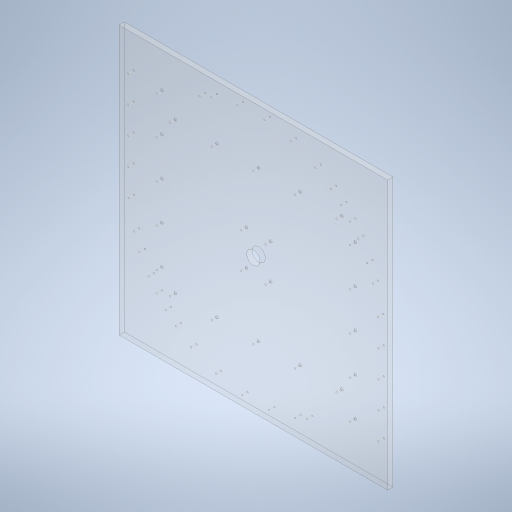
# Autodesk Inventor part: groundPlateWoodV1
Saved by Autodesk Inventor 2024.4 (Build 284460000, 460)
## iProperties
Created: 2025-11-05
Part Number: groundPlateWoodV1
Material: PMMA Plastic
Document SubType Name: Modeling
Designer: jonas
Density: 1.188 g/cm^3
Appearance: Polycarbonate - Clear
Author: jonas
Autodesk Inventor part; units mm, degrees
ref_plane "YZ Plane" through (0, 0, 0) normal (1, 0, 0) x (0, 1, 0)
ref_plane "XZ Plane" through (0, 0, 0) normal (0, 1, 0) x (-1, 0, 0)
ref_plane "XY Plane" through (0, 0, 0) normal (0, 0, 1) x (1, 0, 0)
sketch "Sketch1" plane through (0, 0, 0) normal (0, 1, 0) x (-1, 0, 0)
  line L0 (0, -102.1042) -> (0, 102.1042) construction
  line L1 (37.5532, 0) -> (-37.5532, 0) construction
  line L2 (500, 500) -> (-500, 500)
  line L3 (-500, 500) -> (-500, -500)
  line L4 (-500, -500) -> (500, -500)
  line L5 (500, -500) -> (500, 500)
  circle A0 centre (0, 0) radius 25
  dimension "d0" = 1000
  dimension "d1" = 1000
  dimension "d2" = 50
  constraints: 12 end point, 2 coincident, 2 horizontal, 2 midpoint, 2 parallel, 1 centre point, 1 perpendicular, 1 vertical, 2 other
  measures "d0" distance between parallel lines of L2 L4
  measures "d1" distance between parallel lines of L3 L5
  measures "d2" diameter of A0
extrude "Extrusion1" add sketch "Sketch1" along normal blind 20
sketch "Sketch3" plane through (0, 20, 0) normal (0, 1, 0) x (1, 0, 0)
  line L0 (464.3817, -39.9852) -> (0, 0) construction
  line L1 (0, 0) -> (445.1648, -138.1214) construction
  line L2 (423.7332, -194.1633) -> (0, 0) construction
  line L3 (360.2723, -295.7246) -> (0, 0) construction
  line L4 (289.0138, -365.6778) -> (0, 0) construction
  line L5 (389.8771, -255.4312) -> (0, 0) construction
  line L6 (326.5218, -332.615) -> (0, 0) construction
  line L7 (230.9911, -404.8361) -> (0, 0) construction
  line L8 (139.32, -444.7911) -> (0, 0) construction
  line L9 (41.2359, -464.2723) -> (0, 0) construction
  line L10 (464.3817, -39.9852) -> (445.1648, -138.1214) construction
  line L11 (445.1648, -138.1214) -> (423.7332, -194.1633) construction
  line L12 (423.7332, -194.1633) -> (389.8771, -255.4312) construction
  line L13 (389.8771, -255.4312) -> (360.2723, -295.7246) construction
  line L14 (360.2723, -295.7246) -> (326.5218, -332.615) construction
  line L15 (326.5218, -332.615) -> (289.0138, -365.6778) construction
  line L16 (289.0138, -365.6778) -> (230.9911, -404.8361) construction
  line L17 (230.9911, -404.8361) -> (139.32, -444.7911) construction
  line L18 (139.32, -444.7911) -> (41.2359, -464.2723) construction
  line L19 (-58.7462, -462.3831) -> (0, 0) construction
  line L20 (-156.0243, -439.2102) -> (0, 0) construction
  line L21 (-200, -421.0098) -> (0, 0) construction
  line L22 (41.2359, -464.2723) -> (-58.7462, -462.3831) construction
  line L23 (-58.7462, -462.3831) -> (-156.0243, -439.2102) construction
  line L24 (-200, -421.0098) -> (-156.0243, -439.2102) construction
  line L25 (500, 500) -> (-500, 500) projected
  line L26 (500, -500) -> (500, 500) projected
  line L27 (-16.3542, 0) -> (16.3542, 0) construction
  line L28 (0, 9.5055) -> (0, -9.5055) construction
  line L29 (-500, -500) -> (500, -500) projected
  line L30 (-466.1, -260) -> (-466.1, -360) construction
  line L31 (-500, 500) -> (-500, -500) construction
  line L32 (-466.1, -260) -> (-466.1, -160) construction
  line L33 (-466.1, -160) -> (-466.1, -60) construction
  line L34 (-464.3817, 39.9852) -> (0, 0) construction
  line L35 (-445.1648, 138.1214) -> (0, 0) construction
  circle A0 centre (0, 0) radius 25 construction
  line L36 (-423.7332, 194.1633) -> (0, 0) construction
  line L37 (0, 0) -> (-389.8771, 255.4312) construction
  line L38 (-360.2723, 295.7246) -> (0, 0) construction
  line L39 (-326.5218, 332.615) -> (0, 0) construction
  line L40 (0, 0) -> (-289.0138, 365.6778) construction
  line L41 (-230.9911, 404.8361) -> (0, 0) construction
  line L42 (-139.32, 444.7911) -> (0, 0) construction
  line L43 (-41.2359, 464.2723) -> (0, 0) construction
  line L44 (-466.1, -60) -> (-464.3817, 39.9852) construction
  line L45 (-464.3817, 39.9852) -> (-445.1648, 138.1214) construction
  line L46 (-445.1648, 138.1214) -> (-423.7332, 194.1633) construction
  line L47 (-423.7332, 194.1633) -> (-389.8771, 255.4312) construction
  line L48 (-389.8771, 255.4312) -> (-360.2723, 295.7246) construction
  line L49 (-360.2723, 295.7246) -> (-326.5218, 332.615) construction
  line L50 (-326.5218, 332.615) -> (-289.0138, 365.6778) construction
  line L51 (-289.0138, 365.6778) -> (-230.9911, 404.8361) construction
  line L52 (-230.9911, 404.8361) -> (-139.32, 444.7911) construction
  line L53 (-139.32, 444.7911) -> (-41.2359, 464.2723) construction
  line L54 (58.7462, 462.3831) -> (0, 0) construction
  line L55 (156.0243, 439.2102) -> (0, 0) construction
  line L56 (200, 421.0098) -> (0, 0) construction
  line L57 (58.7462, 462.3831) -> (-41.2359, 464.2723) construction
  line L58 (58.7462, 462.3831) -> (156.0243, 439.2102) construction
  line L59 (156.0243, 439.2102) -> (200, 421.0098) construction
  point P0 (466.1, 360)
  point P1 (466.1, 260)
  point P2 (466.1, 160)
  point P3 (466.1, 60)
  dimension "d62" = 100
  dimension "d63" = 100
  dimension "d64" = 100
  dimension "d66" = 466.1
  dimension "d67" = 100
  dimension "d68" = 100
  dimension "d69" = 60
  dimension "d70" = 70
  dimension "d71" = 50
  dimension "d72" = 70
  dimension "d73" = 100
  dimension "d76" = 140
  dimension "d77" = 33.9
  dimension "d78" = 700
  dimension "d79" = 140
  dimension "d80" = 100
  dimension "d82" = 33.9
  dimension "d84" = 60
  dimension "d85" = 70
  dimension "d86" = 50
  dimension "d87" = 70
  dimension "d88" = 100
  dimension "d89" = 700
  constraints: 112 end point, 39 equal length, 6 vertical alignment, 3 vertical, 2 midpoint, 1 coincident, 1 collinear, 1 horizontal
  measures "d62" distance of point (466.1, 260) point (466.1, 360)
  measures "d63" distance of point (466.1, 260) point (466.1, 160)
  measures "d64" distance of point (466.1, 160) point (466.1, 60)
  measures "d66" distance of L10.start L0.end
  measures "d67" distance of L10.start L11.start
  measures "d68" distance of point (466.1, 60) L10.start
  measures "d69" distance of L11.start L11.end
  measures "d70" distance of L11.end L13.start
  measures "d71" distance of L14.start L14.end
  measures "d72" distance of L17.start L15.end
  measures "d73" distance of L17.start L17.end
  measures "d76" distance from line of L25 point (466.1, 360)
  measures "d77" distance from line of L26 point (466.1, 360)
  measures "d78" distance from line of L26 L24.start
  measures "d79" distance from line of L29 L30.end
  measures "d80" distance of L30.start L30.end
  measures "d82" distance from line of L31 L30.end
  measures "d84" distance of L35.start L36.start
  measures "d85" distance of L36.start L37.end
  measures "d86" distance of L37.end L38.start
  measures "d87" distance of L40.end L41.start
  measures "d88" distance of L41.start L42.start
  measures "d89" distance from line of L31 L56.start
hole "Hole2" at (-200, 20, 421.0098) at (-156.0243, 20, 439.2102) at (-58.7462, 20, 462.3831) at (41.2359, 20, 464.2723) at (139.32, 20, 444.7911) at (230.9911, 20, 404.8361) at (289.0138, 20, 365.6778) at (326.5218, 20, 332.615) at (360.2723, 20, 295.7246) at (389.8771, 20, 255.4312) at (423.7332, 20, 194.1633) at (445.1648, 20, 138.1214) at (464.3817, 20, 39.9852) at (466.1, 20, -60) at (466.1, 20, -160) at (466.1, 20, -260) at (466.1, 20, -360) at (-466.1, 20, 360) at (-466.1, 20, 260) at (-466.1, 20, 160) at (-466.1, 20, 60) at (-464.3817, 20, -39.9852) at (-445.1648, 20, -138.1214) at (-423.7332, 20, -194.1633) at (-389.8771, 20, -255.4312) at (-360.2723, 20, -295.7246) at (-326.5218, 20, -332.615) at (-289.0138, 20, -365.6778) at (-230.9911, 20, -404.8361) at (-139.32, 20, -444.7911) at (-41.2359, 20, -464.2723) at (58.7462, 20, -462.3831) at (156.0243, 20, -439.2102) at (200, 20, -421.0098) direction (0, -1, 0) diameter 5.5 end through all clearance for "Countersunk Flat Head Screw DIN EN ISO 2009" size "M5" standard "DIN"
sketch "Sketch4" plane through (0, 20, 0) normal (0, 1, 0) x (1, 0, 0)
  line L0 (500, -500) -> (500, 500) projected
  line L1 (-500, 500) -> (-500, -500) projected
  line L2 (-500, -500) -> (500, -500) projected
  line L3 (500, 500) -> (-500, 500) projected
  line L4 (-360, 220) -> (-360, 77.5) construction
  line L5 (-360, 77.5) -> (-360, -65) construction
  line L6 (-360, -65) -> (-360, -207.5) construction
  line L7 (-360, -207.5) -> (-360, -350) construction
  line L8 (360, 350) -> (360, 207.5) construction
  line L9 (360, 207.5) -> (360, 65) construction
  line L10 (360, 65) -> (360, -77.5) construction
  line L11 (360, -77.5) -> (360, -220) construction
  line L12 (310, -280) -> (155, -280) construction
  line L13 (155, -280) -> (0, -280) construction
  line L14 (0, -280) -> (-155, -280) construction
  line L15 (-155, -280) -> (-310, -280) construction
  line L16 (-310, 280) -> (-155, 280) construction
  line L17 (-155, 280) -> (0, 280) construction
  line L18 (0, 280) -> (155, 280) construction
  line L19 (155, 280) -> (310, 280) construction
  line L20 (0, 7.0345) -> (0, -7.0345) construction
  line L21 (-9.8826, 0) -> (9.8826, 0) construction
  point P0 (0, 0)
  point P1 (-45, 65)
  point P2 (-45, -65)
  point P3 (45, -65)
  point P4 (45, 65)
  point P5 (0, 0)
  dimension "d42" = 140
  dimension "d43" = 140
  dimension "d44" = 150
  dimension "d45" = 150
  dimension "d46" = 570
  dimension "d47" = 570
  dimension "d55" = 220
  dimension "d56" = 220
  dimension "d57" = 50
  dimension "d58" = 50
  dimension "d59" = 90
  dimension "d60" = 130
  constraints: 36 end point, 24 collinear, 12 vertical alignment, 10 horizontal alignment, 3 horizontal, 3 vertical, 2 midpoint, 2 symmetric about line, 1 coincident
  measures "d42" distance from line of L0 L8.start
  measures "d43" distance from line of L1 L7.end
  measures "d44" distance from line of L2 L7.end
  measures "d45" distance from line of L3 L8.start
  measures "d46" distance of L7.end L4.start
  measures "d47" distance of L8.start L11.end
  measures "d55" distance from line of L12.start L2
  measures "d56" vertical distance of L0.end L19.end
  measures "d57" horizontal distance of L11.end L12.start
  measures "d58" horizontal distance of L7.end L15.end
  measures "d59" distance of point (45, 65) point (-45, 65)
  measures "d60" distance of point (45, -65) point (45, 65)
hole "Hole3" at (360, 20, -350) at (360, 20, -207.5) at (360, 20, 77.5) at (360, 20, 220) at (360, 20, -65) at (-360, 20, 350) at (-360, 20, 207.5) at (-360, 20, 65) at (-360, 20, -220) at (-360, 20, -77.5) at (-310, 20, -280) at (-155, 20, -280) at (0, 20, -280) at (155, 20, -280) at (310, 20, -280) at (310, 20, 280) at (155, 20, 280) at (0, 20, 280) at (-155, 20, 280) at (-310, 20, 280) at (-45, 20, -65) at (45, 20, -65) at (-45, 20, 65) at (45, 20, 65) direction (0, -1, 0) diameter 5.5 end through all countersink diameter 10.4 countersink angle 90 clearance for "Countersunk Flat Head Screw DIN EN ISO 2009" size "M5" standard "DIN"
body "Solid1"
